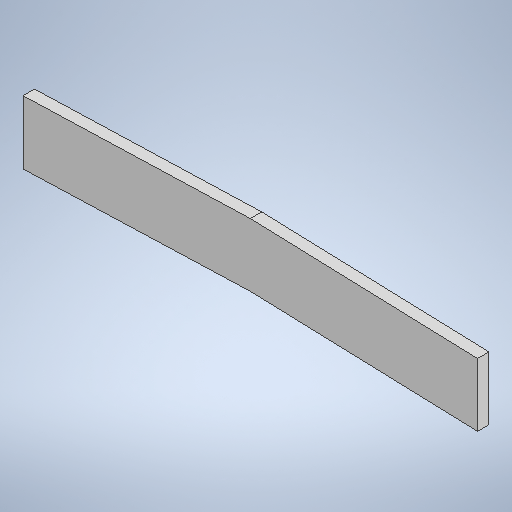
# Autodesk Inventor part: E
Saved by Autodesk Inventor 2025.3 (Build 293356030, 356C)
## iProperties
Created: 2025-07-09
Part Number: E
Material: Generic
Document SubType Name: Modeling
Designer: jv
Density: 1 g/cm^3
Appearance: Default
Author: jv
Autodesk Inventor part; units mm, degrees
ref_plane "YZ Plane" through (0, 0, 0) normal (1, 0, 0) x (0, 1, 0)
ref_plane "XZ Plane" through (0, 0, 0) normal (0, 1, 0) x (-1, 0, 0)
ref_plane "XY Plane" through (0, 0, 0) normal (0, 0, 1) x (1, 0, 0)
sketch "Sketch1" plane through (0, 0, 0) normal (0, 0, 1) x (1, 0, 0)
  line L0 (0, 0) -> (119, 0)
  line L1 (0, 0) -> (0, 16.6)
  line L2 (0, 0) -> (59.5, 0)
  line L3 (59.5, 2) -> (59.5, 18.5)
  line L4 (0, 16.6) -> (59.5, 18.5)
  line L5 (59.5, 2) -> (0, 0)
  line L6 (119, 0) -> (119, 16.5)
  line L7 (59.5, 18.5) -> (119, 16.5)
  line L8 (119, 0) -> (59.5, 2)
  dimension "d0" = 119
  dimension "d1" = 16.6
  dimension "d2" = 59.5
  dimension "d3" = 2
  dimension "d4" = 16.5
  dimension "d5" = 16.5
  constraints: 18 end point, 3 vertical, 1 horizontal, 1 midpoint
  measures "d0" distance of L0.start L0.end
  measures "d1" distance of L0.start L1.end
  measures "d2" horizontal distance of L0.start L3.start
  measures "d3" vertical distance of L0.start L3.start
  measures "d4" distance of L3.start L3.end
  measures "d5" distance of L0.end L6.end
extrude "Extrusion1" add sketch "Sketch1" along normal blind 3 contours L1 L4 L3 L5 | L3 L7 L6 L8
body "Solid1"
